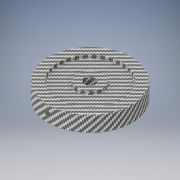
# Autodesk Inventor part: flywheel
Saved by Autodesk Inventor 2017 (Build 210142000, 142)
## iProperties
Created: 2020-01-04
Part Number: flywheel
Material: Steel, Carbon
Document SubType Name: Modeling
Designer: Admin
Density: 7.85 g/cm^3
Appearance: Carbon Fiber
Mass: 124.22 g
Surface Area: 63.0594 cm^2
Volume: 15.8241 cm^3
Author: Admin
Autodesk Inventor part; units mm, degrees
ref_plane "YZ Plane" through (0, 0, 0) normal (1, 0, 0) x (0, 1, 0)
ref_plane "XZ Plane" through (0, 0, 0) normal (0, 1, 0) x (-1, 0, 0)
sketch "Sketch1" plane through (0, 0, 0) normal (0, 1, 0) x (-1, 0, 0)
  circle A0 centre (0, 0) radius 25.4
  circle A1 centre (0, 0) radius 3.175
  dimension "d0" = 50.8
  dimension "d1" = 6.35
  constraints: 2 centre point, 2 coincident
  measures "d0" diameter of A0
  measures "d1" diameter of A1
extrude "Extrusion1" add sketch "Sketch1" along normal mid plane 9.525
sketch "Sketch2" plane through (0, 4.7625, 0) normal (0, 1, 0) x (1, 0, 0)
  circle A0 centre (0, 0) radius 19.05
  circle A1 centre (0, 0) radius 7.9375
  circle A2 centre (0, 0) radius 3.2252
  dimension "d4" = 38.1
  dimension "d5" = 15.875
  constraints: 3 centre point, 3 coincident
  measures "d4" diameter of A0
  measures "d5" diameter of A1
extrude "Extrusion2" cut sketch "Sketch2" against normal blind 1.5875 contours A0
sketch "Sketch3" plane through (0, -4.7625, 0) normal (0, -1, 0) x (1, 0, 0)
  circle A0 centre (0, 0) radius 19.05
  circle A1 centre (0, 0) radius 7.9375
  dimension "d8" = 38.1
  dimension "d9" = 15.875
  constraints: 2 centre point, 2 coincident
  measures "d8" diameter of A0
  measures "d9" diameter of A1
extrude "Extrusion3" cut sketch "Sketch3" against normal blind 1.5875
ref_plane "Work Plane1" through (0, 0, 25.4) normal (0, 0, 1) x (1, 0, 0)
sketch "Sketch4" plane through (0, 0, 25.4) normal (0, 0, 1) x (1, 0, 0)
  circle A0 centre (0, 0) radius 1.7975
  constraints: 1 centre point, 1 coincident
hole "Hole1" at (0, 0, 25.4) direction (0, 0, -1) diameter 3.302 depth 5.9436 tip angle 118 thread size "8-32 UNC" class "2B" standard "ANSI Unified Screw Threads"
sketch "Sketch5" plane through (0, 0, 25.4) normal (0, 0, 1) x (1, 0, 0)
  circle A0 centre (0, 0) radius 1.5875
  dimension "d28" = 3.175
  constraints: 1 centre point, 1 coincident
  measures "d28" diameter of A0
hole "Hole2" at (0, 0, 25.4) direction (0, 0, -1) diameter 3.175 depth 23.4061 tip angle 118
fillet "Fillet1" radius 0.3175 13 edges at (3.175, 4.7625, 0) (-7.9375, 4.7625, 0) (-7.9375, 3.175, 0) (-19.05, 3.175, 0) (-7.9375, -3.175, 0) (-19.05, -3.175, 0) (25.4, -4.7625, 0) (25.4, 4.7625, 0) (3.175, -4.7625, 0) (0, 1.651, 19.4564) (0.0011, 1.5875, 3.175) (-19.05, 4.7625, 0) (-19.05, -4.7625, 0)
fillet "Fillet2" radius 0.3175 1 edges at (-7.9375, -4.7625, 0)
extrude "Extrusion4" add sketch "Sketch5" against normal blind 22.225
hole "Hole3" at (0, 0, 25.4) direction (0, 0, -1) diameter 3.302 depth 6.35 tip angle 118 thread size "8-32 UNC" class "2B" standard "ANSI Unified Screw Threads"
body "Solid1"
